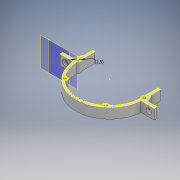
# Autodesk Inventor part: anneau
Saved by Autodesk Inventor 2017 (Build 210142000, 142)
## iProperties
Part Number: anneau
Material: Générique
Document SubType Name: Modeling
Designer: Thomas
Density: 1 g/cm^3
Appearance: Par défaut
Author: Thomas
Autodesk Inventor part; units mm, degrees
ref_plane "YZ Plane" through (0, 0, 0) normal (1, 0, 0) x (0, 1, 0)
ref_plane "XZ Plane" through (0, 0, 0) normal (0, 1, 0) x (-1, 0, 0)
ref_plane "XY Plane" through (0, 0, 0) normal (0, 0, 1) x (1, 0, 0)
sketch "Esquisse1" plane through (0, 0, 0) normal (0, 0, 1) x (1, 0, 0)
  line L0 (0, 0) -> (-27.546, -25.0426) construction
  line L1 (0, 0) -> (23.0277, -27.4577) construction
  circle A0 centre (-18.0975, -16.4528) radius 1.25
  circle A1 centre (15.7127, -18.7355) radius 1.25
  arc A2 (-16.6894, -17.8731) -> (14.1299, -19.9581) centre (0, 0) ccw
  arc A3 (-16.6894, -17.8731) -> (-19.3824, -14.9201) centre (-18.0975, -16.4528) ccw
  arc A4 (17.0433, -17.2424) -> (14.1299, -19.9581) centre (15.7127, -18.7355) ccw
  line L2 (0, 0) -> (-29.5508, 10.7556) construction
  line L3 (-17.8311, 0) -> (17.1748, 0) construction
  line L4 (0, 2.0526) -> (0, -2.2236) construction
  line L5 (-28.8657, 0) -> (-36, 0)
  line L6 (28.8657, 0) -> (36, 0)
  line L7 (36, 0) -> (36, -2)
  line L8 (36, -2) -> (25.923, -2)
  line L9 (-36, 0) -> (-36, -2)
  line L10 (-36, -2) -> (-25.923, -2)
  arc A5 (-25.923, -2) -> (25.923, -2) centre (0, 0) ccw
  circle A6 centre (0, 0) radius 22.5 construction
  arc A7 (-16.6894, -17.8731) -> (14.1299, -19.9581) centre (0, 0) ccw
  arc A8 (-16.6894, -17.8731) -> (14.1299, -19.9581) centre (0, 0) ccw
  circle A9 centre (-25.3169, 1.1605) radius 1.25
  circle A10 centre (25.3169, 1.1605) radius 1.25
  line L11 (24.0891, 2.7784) -> (24.0891, 12.8348)
  line L12 (25.8363, 12.8348) -> (24.0891, 12.8348)
  line L13 (-25.923, 6.143) -> (-25.923, 12.7847)
  line L14 (-24.2942, 2.9148) -> (-24.2942, 12.7847)
  line L15 (-24.2942, 12.7847) -> (-25.923, 12.7847)
  arc A11 (-24.4506, -0.676) -> (-19.3824, -14.9201) centre (0, 0) ccw
  arc A12 (-24.4506, -0.676) -> (-19.3824, -14.9201) centre (0, 0) ccw
  arc A13 (-24.4506, -0.676) -> (-24.2942, 2.9148) centre (-25.3169, 1.1605) ccw
  arc A14 (17.0433, -17.2424) -> (24.2376, -0.5599) centre (0, 0) ccw
  arc A15 (17.0433, -17.2424) -> (24.2376, -0.5599) centre (0, 0) ccw
  arc A16 (17.0433, -17.2424) -> (24.2376, -0.5599) centre (0, 0) ccw
  arc A17 (24.0891, 2.7784) -> (24.2376, -0.5599) centre (25.3169, 1.1605) ccw
  line L16 (-28.8657, 0) -> (-25.923, 6.143)
  line L17 (28.8657, 0) -> (25.923, 6.143)
  line L18 (25.8363, 3.0919) -> (25.8363, 3.124)
  line L19 (25.8363, 6.3239) -> (25.8363, 12.8348)
  line L20 (25.8363, 6.3239) -> (28.8657, 0)
  point P0 (-26.3114, 9.5766)
  dimension "d35" = 2.5
  dimension "d36" = 2.5
  dimension "d37" = 4
  dimension "d38" = 4
  dimension "d39" = 20
  dimension "d44" = 2
  dimension "d45" = 2
  dimension "d52" = 45
  dimension "d65" = 2.5
  constraints: 42 end point, 27 point on circle, 18 centre point, 7 coincident, 6 point on line, 6 vertical, 4 perpendicular, 4 symmetric about line, 3 horizontal, 1 other
  measures "d35" diameter of A0
  measures "d36" diameter of A1
  measures "d37" diameter of A3
  measures "d38" diameter of A4
  measures "d39" angle of L3 L2
  measures "d44" distance of L6.end L7.end
  measures "d45" distance of L5.end L9.end
  measures "d52" diameter of A6
  measures "d65" diameter of A9
ref_plane "Plan de construction1" through (-42, 0, 0) normal (0, 1, 0) x (1, 0, 0)
ref_plane "Plan de construction2" through (-36, 0, 0) normal (0, 1, 0) x (1, 0, 0)
sketch "Esquisse3" plane through (-36, 0, 0) normal (0, 1, 0) x (1, 0, 0)
  line L0 (0, 0) -> (10, 0) projected
  line L1 (0, 0) -> (0, -8) projected
  line L2 (10, -8) -> (0, -8) projected
  line L3 (10, 0) -> (10, -8) projected
  circle A0 centre (4, -4) radius 2.15
  line L4 (62, 0) -> (72, 0) projected
  line L5 (62, 0) -> (62, -8) projected
  line L6 (72, -8) -> (62, -8) projected
  line L7 (72, 0) -> (72, -8) projected
  circle A1 centre (68, -4) radius 2.15
  point P0 (36, 0)
  dimension "d48" = 4.3
  dimension "d73" = 4
  dimension "d74" = 4.3
  dimension "d75" = 4
  constraints: 2 centre point
  measures "d48" diameter of A0
  measures "d73" distance from line of L1 A0.centre
  measures "d74" diameter of A1
  measures "d75" distance from line of L7 A1.centre
extrude "Extrusion14" add sketch "Esquisse1" along normal blind 8
extrude "Extrusion15" cut sketch "Esquisse3" against normal blind 8 contours A0 | A1
sketch "Esquisse4" plane through (0, 0, 8) normal (0, 0, 1) x (1, 0, 0)
  circle A0 centre (25.3169, 1.1605) radius 1.25 projected
  circle A1 centre (-25.3169, 1.1605) radius 1.25 projected
  circle A2 centre (15.7127, -18.7355) radius 1.25 projected
  circle A3 centre (-18.0975, -16.4528) radius 1.25 projected
  arc A4 (-16.6894, -17.8731) -> (-19.3824, -14.9201) centre (-18.0975, -16.4528) ccw projected
  arc A5 (-24.4506, -0.676) -> (-19.3824, -14.9201) centre (0, 0) ccw projected
  arc A6 (-24.4506, -0.676) -> (-24.2942, 2.9148) centre (-25.3169, 1.1605) ccw projected
  line L0 (-24.2942, 2.9148) -> (-24.2942, 12.7847) projected
  line L1 (-24.2942, 12.7847) -> (-25.923, 12.7847) projected
  line L2 (-25.923, 12.7847) -> (-25.923, 6.143) projected
  line L3 (-25.923, 6.143) -> (-28.8657, 0) projected
  line L4 (-28.8657, 0) -> (-36, 0) projected
  line L5 (-36, 0) -> (-36, -2) projected
  line L6 (-36, -2) -> (-25.923, -2) projected
  arc A7 (-25.923, -2) -> (25.923, -2) centre (0, 0) ccw projected
  line L7 (25.923, -2) -> (36, -2) projected
  line L8 (36, -2) -> (36, 0) projected
  line L9 (36, 0) -> (28.8657, 0) projected
  line L10 (28.8657, 0) -> (25.8363, 6.3239) projected
  line L11 (25.8363, 6.3239) -> (25.8363, 12.8348) projected
  line L12 (25.8363, 12.8348) -> (24.0891, 12.8348) projected
  line L13 (24.0891, 12.8348) -> (24.0891, 2.7784) projected
  arc A8 (24.0891, 2.7784) -> (24.2376, -0.5599) centre (25.3169, 1.1605) ccw projected
  arc A9 (17.0433, -17.2424) -> (24.2376, -0.5599) centre (0, 0) ccw projected
  arc A10 (17.0433, -17.2424) -> (14.1299, -19.9581) centre (15.7127, -18.7355) ccw projected
  arc A11 (-16.6894, -17.8731) -> (14.1299, -19.9581) centre (0, 0) ccw projected
  dimension "d78" = 2.5
  measures "d78" diameter of A1
